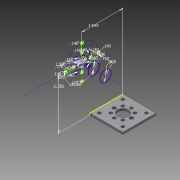
# Autodesk Inventor part: Channel Bracket B
Saved by Autodesk Inventor 2014 SP1 (Build 180222100, 222)
## iProperties
Created: 2014-01-22
Part Number: Channel Bracket B
Material: Generic
Document SubType Name: Modeling
Designer: tom
Density: 1 g/cm^3
Appearance: Default
Author: tom
Autodesk Inventor part; units mm, degrees
ref_plane "YZ Plane" through (0, 0, 0) normal (1, 0, 0) x (0, 1, 0)
ref_plane "XZ Plane" through (0, 0, 0) normal (0, 1, 0) x (-1, 0, 0)
ref_plane "XY Plane" through (0, 0, 0) normal (0, 0, 1) x (1, 0, 0)
sketch "Sketch1" plane through (0, 0, 0) normal (0, 1, 0) x (-1, 0, 0)
  line L0 (-19.05, 19.05) -> (19.05, 19.05)
  line L1 (19.05, 19.05) -> (19.05, -19.05)
  line L2 (19.05, -19.05) -> (-19.05, -19.05)
  line L3 (-19.05, -19.05) -> (-19.05, 19.05)
  circle A0 centre (0, 0) radius 6.35
  circle A1 centre (0, 0) radius 19.05 construction
  circle A2 centre (0, 0) radius 9.779 construction
  line L4 (19.05, -19.05) -> (-19.05, 19.05) construction
  line L5 (19.05, 19.05) -> (-19.05, -19.05) construction
  circle A3 centre (0, -9.779) radius 1.778
  circle A4 centre (6.9148, -6.9148) radius 1.778
  circle A5 centre (-6.9148, -6.9148) radius 1.778
  circle A6 centre (-6.9148, 6.9148) radius 1.778
  circle A7 centre (0, 9.779) radius 1.778
  circle A8 centre (6.9148, 6.9148) radius 1.778
  circle A9 centre (-9.779, 0) radius 2.032
  circle A10 centre (9.779, 0) radius 2.032
  circle A11 centre (-13.4704, 13.4704) radius 1.778
  circle A12 centre (13.4704, 13.4704) radius 1.778
  circle A13 centre (13.4704, -13.4704) radius 1.778
  circle A14 centre (-13.4704, -13.4704) radius 1.778
  dimension "d5" = 19.558
  dimension "d0" = 19.05
  dimension "d1" = 38.1
  dimension "d2" = 38.1
  dimension "d3" = 19.05
  dimension "d4" = 12.7
  dimension "d6" = 3.556
  dimension "d7" = 3.556
  dimension "d8" = 3.556
  dimension "d9" = 3.556
  dimension "d10" = 3.556
  dimension "d11" = 3.556
  dimension "d12" = 4.064
  dimension "d13" = 4.064
  dimension "d14" = 3.556
  dimension "d15" = 3.556
  dimension "d16" = 3.556
  dimension "d17" = 3.556
  constraints: 14 centre point, 12 end point, 9 point on line, 4 point on circle, 3 coincident, 2 parallel, 2 perpendicular, 1 horizontal, 10 other
  measures "d0" distance from line of L3 point (0, 0)
  measures "d1" distance between parallel lines of L1 L3
  measures "d2" distance of L0.end L1.end
  measures "d3" distance from line of L2 point (0, 0)
  measures "d4" diameter of A0
  measures "d6" diameter of A3
  measures "d7" diameter of A4
  measures "d8" diameter of A5
  measures "d9" diameter of A6
  measures "d10" diameter of A7
  measures "d11" diameter of A8
  measures "d12" diameter of A9
  measures "d13" diameter of A10
  measures "d14" diameter of A11
  measures "d15" diameter of A12
  measures "d16" diameter of A13
  measures "d17" diameter of A14
extrude "Extrusion1" add sketch "Sketch1" along normal blind 2.286
sketch "Sketch2" plane through (-19.05, 0, -19.05) normal (-1, 0, 0) x (0, 0, 1)
  line L0 (38.1, 0) -> (0, 0) projected
  line L1 (38.1, 0) -> (38.1, 2.286) projected
  line L2 (0, 2.286) -> (38.1, 2.286) projected
  line L3 (0, 0) -> (0, 2.286) projected
  circle A0 centre (46.9646, 57.15) radius 6.35
  line L4 (46.9646, 57.15) -> (0, 10.1854) construction
  line L5 (46.9646, 57.15) -> (113.3826, 57.15) construction
  circle A1 centre (33.4942, 43.6796) radius 6.35
  circle A2 centre (20.0238, 30.2092) radius 6.35
  circle A3 centre (46.9646, 57.15) radius 9.779 construction
  circle A4 centre (46.9646, 57.15) radius 19.05 construction
  line L6 (42.4745, 52.6599) -> (60.435, 70.6204) construction
  line L7 (46.9646, 57.15) -> (60.4393, 57.15) construction
  line L8 (60.435, 43.6796) -> (33.4942, 70.6204) construction
  line L9 (46.9646, 57.15) -> (60.4393, 57.15) construction
  line L10 (27.9146, 57.15) -> (66.0146, 57.15) construction
  circle A5 centre (40.0498, 64.0648) radius 1.778
  circle A6 centre (46.9646, 66.929) radius 1.778
  circle A7 centre (37.1856, 57.15) radius 1.778
  circle A8 centre (46.9646, 47.371) radius 1.778
  circle A9 centre (53.8794, 50.2352) radius 1.778
  circle A10 centre (56.7436, 57.15) radius 1.778
  circle A11 centre (53.8794, 64.0648) radius 2.032
  circle A12 centre (40.0498, 50.2352) radius 2.032
  circle A13 centre (46.9646, 76.2) radius 1.778
  circle A14 centre (27.9146, 57.15) radius 1.778
  circle A15 centre (46.9646, 38.1) radius 1.778
  circle A16 centre (66.0146, 57.15) radius 1.778
  point P0 (19.05, 0)
  dimension "d20" = 12.7
  dimension "d28" = 19.558
  dimension "d29" = 38.1
  dimension "d21" = 57.15
  dimension "d22" = 46.9646
  dimension "d23" = 135
  dimension "d24" = 12.7
  dimension "d25" = 19.05
  dimension "d26" = 12.7
  dimension "d27" = 19.05
  dimension "d30" = 45
  dimension "d31" = 135
  dimension "d32" = 3.556
  dimension "d33" = 3.556
  dimension "d34" = 3.556
  dimension "d35" = 3.556
  dimension "d36" = 3.556
  dimension "d37" = 3.556
  dimension "d38" = 4.064
  dimension "d39" = 4.064
  dimension "d40" = 3.556
  dimension "d41" = 3.556
  dimension "d42" = 3.556
  dimension "d43" = 3.556
  constraints: 14 centre point, 14 end point, 9 point on line, 4 coincident, 3 horizontal, 1 equal length, 1 midpoint, 22 other
  measures "d21" distance from line of L4.start L0
  measures "d22" distance from line of L3 L4.start
  measures "d23" angle of L4 L5
  measures "d24" diameter of A1
  measures "d25" distance of A1.centre L4.start
  measures "d26" diameter of A2
  measures "d27" distance of A2.centre A1.centre
  measures "d30" angle of L7 L6
  measures "d31" angle of L9 L8
  measures "d32" diameter of A5
  measures "d33" diameter of A6
  measures "d34" diameter of A7
  measures "d35" diameter of A8
  measures "d36" diameter of A9
  measures "d37" diameter of A10
  measures "d38" diameter of A11
  measures "d39" diameter of A12
  measures "d40" diameter of A13
  measures "d41" diameter of A14
  measures "d42" diameter of A15
  measures "d43" diameter of A16
body "Solid1"
